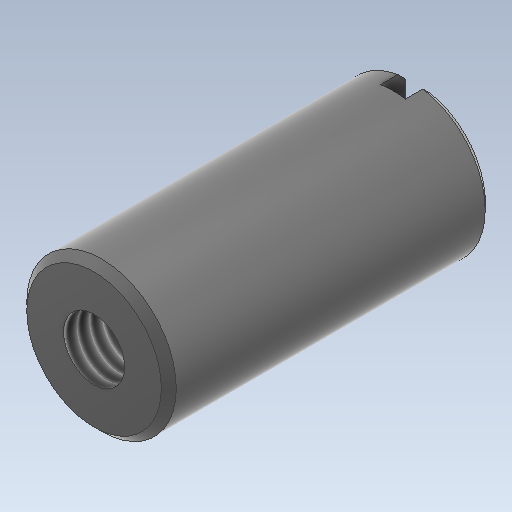
# Autodesk Inventor part: ARL-313SBE
Saved by Autodesk Inventor 2020.3 (Build 243373000, 373)
## iProperties
Created: 2021-06-02
Part Number: ARL-313SBE
Material: アルミニウム 2014-T4
Document SubType Name: Modeling
Designer: masato
Density: 2.8 g/cm^3
Appearance: 滑らか - 黒
Author: masato
Autodesk Inventor part; units mm, degrees
ref_plane "YZ Plane" through (0, 0, 0) normal (1, 0, 0) x (0, 1, 0)
ref_plane "XZ Plane" through (0, 0, 0) normal (0, 1, 0) x (-1, 0, 0)
ref_plane "XY Plane" through (0, 0, 0) normal (0, 0, 1) x (1, 0, 0)
sketch "スケッチ1" plane through (0, 0, 0) normal (0, 0, 1) x (1, 0, 0)
  circle A0 centre (0, 0) radius 3
  line L0 (0, 3) -> (0, -3) construction
  line L1 (-0.5, 2.958) -> (-0.5, -2.958)
  line L2 (0.5, 2.958) -> (0.5, -2.958)
  dimension "d0" = 6
  dimension "d1" = 1
  constraints: 6 end point, 4 point on circle, 2 coincident, 2 symmetric about line, 2 vertical, 1 centre point, 1 midpoint
  measures "d0" diameter of A0
  measures "d1" distance between parallel lines of L2 L1
extrude "押し出し1" add sketch "スケッチ1" along normal blind 13
extrude "押し出し2" cut sketch "スケッチ1" along normal blind 1 contours L2 A0 L1
chamfer "面取り1" distance 0.3 angle 45 4 edges at (-3, 0, 13) (2.2913, 1.9365, 0) (2.2913, -1.9365, 0) (-3, 0, 0)
hole "穴1" at (0, 0, 0) direction (0, 0, 1) diameter 2.459 end through all thread size "M3x0.5" class "6H" standard "ISO Metric profile"
